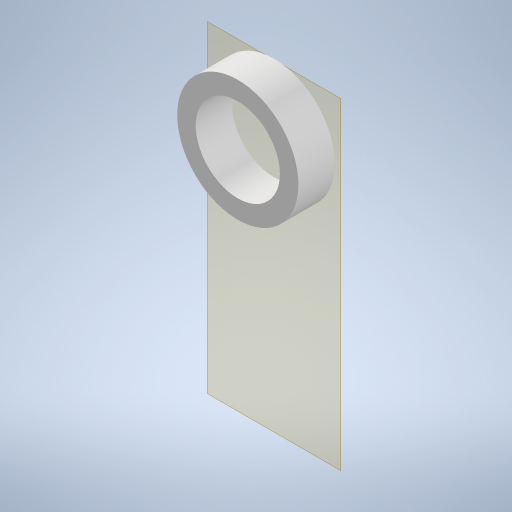
# Autodesk Inventor part: spacerA_V3
Saved by Autodesk Inventor 2023 (Build 270158000, 158)
## iProperties
Created: 2022-11-25
Part Number: spacerA_V3
Material: Generic
Document SubType Name: Modeling
Designer: shrey
Density: 1 g/cm^3
Appearance: Default
Author: shrey
Autodesk Inventor part; units mm, degrees
(part 1 of 2)
ref_plane "YZ Plane" through (0, 0, 0) normal (1, 0, 0) x (0, 1, 0)
ref_plane "XZ Plane" through (0, 0, 0) normal (0, 1, 0) x (-1, 0, 0)
ref_plane "XY Plane" through (0, 0, 0) normal (0, 0, 1) x (1, 0, 0)
ref_plane "Work Plane1" through (-7.7432, -45.9796, 22.0468) normal (0, 0, 1) x (1, 0, 0)
sketch "Sketch1" plane through (-7.7432, -45.9796, 22.0468) normal (0, 0, 1) x (1, 0, 0)
  spline S0 degree 3 poles (3.2142, 51.1538) (3.1859, 51.0451) (3.1294, 50.8276) (3.0543, 50.4989) (2.9867, 50.1686) (2.9278, 49.8367) (2.8779, 49.5033) (2.8377, 49.1686) (2.808, 48.8328) (2.7898, 48.4962) (2.7854, 48.2152) (2.7893, 47.9905) (2.7963, 47.8221) (2.8075, 47.6539) (2.8251, 47.4863) (2.8413, 47.3468) (2.8467, 47.2345) (2.846, 47.1502) (2.8418, 47.066) (2.8328, 46.9822) (2.8184, 46.8991) (2.7981, 46.8172) (2.7715, 46.7372) (2.7385, 46.6595) (2.6988, 46.5851) (2.6518, 46.5149) (2.5985, 46.4496) (2.5398, 46.389) (2.4742, 46.3358) (2.4039, 46.2892) (2.3294, 46.2495) (2.2239, 46.2102) (2.0895, 46.1697) (1.9569, 46.1234) (1.8485, 46.0931) (1.7649, 46.0814) (1.6806, 46.0777) (1.5963, 46.0822) (1.5132, 46.0968) (1.4316, 46.1182) (1.3524, 46.1473) (1.2765, 46.1842) (1.2041, 46.2275) (1.1356, 46.2767) (1.071, 46.3309) (1.0104, 46.3896) (0.9538, 46.4521) (0.901, 46.5178) (0.8509, 46.5856) (0.7892, 46.6795) (0.7202, 46.8019) (0.6359, 46.9478) (0.546, 47.0905) (0.4527, 47.2308) (0.3236, 47.4148) (0.1549, 47.6395) (-0.0578, 47.901) (-0.2793, 48.1552) (-0.5087, 48.4022) (-0.7451, 48.6425) (-0.988, 48.8763) (-1.2369, 49.1037) (-1.4909, 49.3254) (-1.6645, 49.468) (-1.7513, 49.5393) knots -1.078574 -1.078574 -1.078574 -1.078574 -1.044867 -1.011159 -0.977452 -0.943745 -0.910038 -0.876331 -0.842624 -0.808918 -0.775212 -0.758359 -0.741505 -0.724651 -0.707798 -0.690947 -0.68252 -0.674093 -0.665668 -0.657242 -0.648815 -0.640389 -0.631963 -0.623537 -0.61511 -0.606685 -0.598264 -0.589839 -0.581413 -0.57299 -0.564565 -0.556141 -0.539287 -0.522433 -0.514009 -0.505584 -0.49716 -0.488735 -0.48031 -0.471889 -0.463464 -0.455037 -0.446611 -0.438185 -0.429758 -0.421332 -0.412906 -0.40448 -0.396053 -0.387627 -0.370775 -0.353922 -0.337069 -0.320215 -0.303361 -0.269656 -0.235949 -0.202243 -0.168536 -0.134829 -0.101122 -0.067415 -0.033707 0 0 0 0 construction
  arc A0 (-1.7513, 49.5393) -> (-3.0984, 48.9393) centre (10.5928, 20.0161) ccw construction
  spline S1 degree 3 poles (-3.0984, 48.9393) (-3.1035, 48.827) (-3.1136, 48.6025) (-3.1187, 48.2654) (-3.1161, 47.9283) (-3.1047, 47.5914) (-3.0843, 47.2549) (-3.054, 46.9192) (-3.0132, 46.5845) (-2.961, 46.2515) (-2.9069, 45.9757) (-2.8564, 45.7568) (-2.8145, 45.5935) (-2.7686, 45.4313) (-2.7165, 45.271) (-2.6717, 45.1379) (-2.6431, 45.0292) (-2.6262, 44.9466) (-2.6128, 44.8634) (-2.6041, 44.7795) (-2.601, 44.6952) (-2.6039, 44.6109) (-2.6132, 44.5271) (-2.6293, 44.4443) (-2.6527, 44.3632) (-2.6841, 44.2849) (-2.7227, 44.2099) (-2.7674, 44.1383) (-2.8205, 44.0727) (-2.8796, 44.0125) (-2.9443, 43.9582) (-3.0393, 43.8979) (-3.1623, 43.8302) (-3.2824, 43.7574) (-3.3821, 43.7052) (-3.4615, 43.6764) (-3.5432, 43.6553) (-3.6266, 43.6421) (-3.7109, 43.6391) (-3.7951, 43.6431) (-3.8787, 43.6551) (-3.9606, 43.6753) (-4.0404, 43.7027) (-4.1177, 43.7366) (-4.1921, 43.7762) (-4.2635, 43.821) (-4.3319, 43.8704) (-4.3973, 43.9236) (-4.4604, 43.9795) (-4.5403, 44.0586) (-4.6332, 44.164) (-4.746, 44.2892) (-4.8635, 44.41) (-4.984, 44.5279) (-5.1485, 44.681) (-5.3603, 44.8656) (-5.6227, 45.0773) (-5.8922, 45.2798) (-6.1679, 45.4738) (-6.4491, 45.6597) (-6.7353, 45.8379) (-7.026, 46.0085) (-7.3205, 46.1726) (-7.5201, 46.276) (-7.6198, 46.3277) knots -1.078574 -1.078574 -1.078574 -1.078574 -1.044867 -1.011159 -0.977452 -0.943745 -0.910038 -0.876331 -0.842624 -0.808918 -0.775212 -0.758359 -0.741505 -0.724651 -0.707798 -0.690947 -0.68252 -0.674093 -0.665668 -0.657242 -0.648815 -0.640389 -0.631963 -0.623537 -0.61511 -0.606685 -0.598264 -0.589839 -0.581413 -0.57299 -0.564565 -0.556141 -0.539287 -0.522433 -0.514009 -0.505584 -0.49716 -0.488735 -0.48031 -0.471889 -0.463464 -0.455037 -0.446611 -0.438185 -0.429758 -0.421332 -0.412906 -0.40448 -0.396053 -0.387627 -0.370775 -0.353922 -0.337069 -0.320215 -0.303361 -0.269656 -0.235949 -0.202243 -0.168536 -0.134829 -0.101122 -0.067415 -0.033707 0 0 0 0 construction
  arc A1 (-7.6198, 46.3277) -> (-8.8127, 45.4607) centre (10.5928, 20.0161) ccw construction
  spline S2 degree 3 poles (-8.8127, 45.4607) (-8.7943, 45.3498) (-8.7575, 45.1281) (-8.6924, 44.7973) (-8.6198, 44.4682) (-8.5387, 44.141) (-8.4487, 43.8161) (-8.3492, 43.494) (-8.2398, 43.1751) (-8.1195, 42.8602) (-8.0092, 42.6017) (-7.9143, 42.398) (-7.8394, 42.247) (-7.7607, 42.0979) (-7.6765, 41.952) (-7.6049, 41.8311) (-7.5543, 41.7307) (-7.5207, 41.6534) (-7.4902, 41.5748) (-7.4644, 41.4946) (-7.4438, 41.4128) (-7.429, 41.3297) (-7.4207, 41.2458) (-7.4193, 41.1614) (-7.4253, 41.0773) (-7.4397, 40.9941) (-7.4619, 40.9128) (-7.4908, 40.8335) (-7.529, 40.7582) (-7.5743, 40.687) (-7.6263, 40.6205) (-7.7067, 40.5417) (-7.813, 40.45) (-7.9153, 40.3538) (-8.002, 40.282) (-8.0736, 40.2373) (-8.1491, 40.1997) (-8.228, 40.1694) (-8.3098, 40.149) (-8.3931, 40.1354) (-8.4773, 40.1297) (-8.5616, 40.1325) (-8.6453, 40.1427) (-8.728, 40.1597) (-8.809, 40.183) (-8.8882, 40.212) (-8.9653, 40.2461) (-9.0403, 40.2846) (-9.1137, 40.3261) (-9.2083, 40.3868) (-9.3211, 40.4706) (-9.4575, 40.5696) (-9.5975, 40.6634) (-9.7399, 40.7536) (-9.9326, 40.8692) (-10.1782, 41.0058) (-10.4788, 41.1583) (-10.7846, 41.3003) (-11.0946, 41.4327) (-11.4083, 41.5561) (-11.7253, 41.6709) (-12.0451, 41.7774) (-12.3673, 41.8766) (-12.584, 41.9363) (-12.6923, 41.9661) knots -1.078574 -1.078574 -1.078574 -1.078574 -1.044867 -1.011159 -0.977452 -0.943745 -0.910038 -0.876331 -0.842624 -0.808918 -0.775212 -0.758359 -0.741505 -0.724651 -0.707798 -0.690947 -0.68252 -0.674093 -0.665668 -0.657242 -0.648815 -0.640389 -0.631963 -0.623537 -0.61511 -0.606685 -0.598264 -0.589839 -0.581413 -0.57299 -0.564565 -0.556141 -0.539287 -0.522433 -0.514009 -0.505584 -0.49716 -0.488735 -0.48031 -0.471889 -0.463464 -0.455037 -0.446611 -0.438185 -0.429758 -0.421332 -0.412906 -0.40448 -0.396053 -0.387627 -0.370775 -0.353922 -0.337069 -0.320215 -0.303361 -0.269656 -0.235949 -0.202243 -0.168536 -0.134829 -0.101122 -0.067415 -0.033707 0 0 0 0 construction
  arc A2 (-12.6923, 41.9661) -> (-13.6789, 40.87) centre (10.5928, 20.0161) ccw construction
  spline S3 degree 3 poles (-13.6789, 40.87) (-13.6378, 40.7654) (-13.5558, 40.5562) (-13.4233, 40.2462) (-13.2838, 39.9393) (-13.1364, 39.6361) (-12.9808, 39.337) (-12.8166, 39.0426) (-12.6433, 38.7535) (-12.4601, 38.4705) (-12.2985, 38.2406) (-12.1634, 38.0611) (-12.0587, 37.929) (-11.9507, 37.7995) (-11.838, 37.6742) (-11.7428, 37.5709) (-11.6725, 37.4832) (-11.6235, 37.4146) (-11.5774, 37.344) (-11.5354, 37.2709) (-11.4983, 37.1952) (-11.4666, 37.117) (-11.441, 37.0366) (-11.4221, 36.9544) (-11.4104, 36.8709) (-11.4072, 36.7865) (-11.412, 36.7023) (-11.4238, 36.6188) (-11.4456, 36.5372) (-11.4751, 36.4582) (-11.512, 36.3822) (-11.5743, 36.2885) (-11.6592, 36.1766) (-11.7393, 36.0613) (-11.8092, 35.9731) (-11.87, 35.9144) (-11.936, 35.8619) (-12.0068, 35.816) (-12.0826, 35.7789) (-12.1612, 35.7483) (-12.2424, 35.7253) (-12.3255, 35.7105) (-12.4095, 35.7031) (-12.4939, 35.7025) (-12.578, 35.7085) (-12.6615, 35.7204) (-12.744, 35.7377) (-12.8254, 35.7597) (-12.9057, 35.7851) (-13.0109, 35.8248) (-13.1386, 35.8833) (-13.2926, 35.9518) (-13.4491, 36.0144) (-13.6071, 36.0731) (-13.8197, 36.1461) (-14.0883, 36.2286) (-14.4141, 36.3152) (-14.7427, 36.3906) (-15.0734, 36.4557) (-15.406, 36.5111) (-15.7399, 36.5575) (-16.0749, 36.5951) (-16.4106, 36.6252) (-16.635, 36.6385) (-16.7471, 36.6452) knots -1.078574 -1.078574 -1.078574 -1.078574 -1.044867 -1.011159 -0.977452 -0.943745 -0.910038 -0.876331 -0.842624 -0.808918 -0.775212 -0.758359 -0.741505 -0.724651 -0.707798 -0.690947 -0.68252 -0.674093 -0.665668 -0.657242 -0.648815 -0.640389 -0.631963 -0.623537 -0.61511 -0.606685 -0.598264 -0.589839 -0.581413 -0.57299 -0.564565 -0.556141 -0.539287 -0.522433 -0.514009 -0.505584 -0.49716 -0.488735 -0.48031 -0.471889 -0.463464 -0.455037 -0.446611 -0.438185 -0.429758 -0.421332 -0.412906 -0.40448 -0.396053 -0.387627 -0.370775 -0.353922 -0.337069 -0.320215 -0.303361 -0.269656 -0.235949 -0.202243 -0.168536 -0.134829 -0.101122 -0.067415 -0.033707 0 0 0 0 construction
  arc A3 (-16.7471, 36.6452) -> (-17.4843, 35.3679) centre (10.5928, 20.0161) ccw construction
  spline S4 degree 3 poles (-17.4843, 35.3679) (-17.4224, 35.2741) (-17.2986, 35.0866) (-17.1045, 34.8109) (-16.9043, 34.5397) (-16.6971, 34.2738) (-16.4828, 34.0136) (-16.2609, 33.7598) (-16.0312, 33.513) (-15.7932, 33.2742) (-15.5874, 33.083) (-15.4178, 32.9355) (-15.288, 32.828) (-15.1555, 32.7238) (-15.0191, 32.6247) (-14.9046, 32.5434) (-14.8176, 32.4722) (-14.7554, 32.4154) (-14.6956, 32.3559) (-14.6393, 32.2931) (-14.5872, 32.2268) (-14.54, 32.1569) (-14.4983, 32.0836) (-14.4627, 32.0071) (-14.4339, 31.9278) (-14.4132, 31.846) (-14.4004, 31.7626) (-14.3946, 31.6785) (-14.3989, 31.5941) (-14.4113, 31.5107) (-14.4317, 31.4287) (-14.4731, 31.3241) (-14.5329, 31.197) (-14.5873, 31.0675) (-14.6373, 30.9668) (-14.6845, 30.8967) (-14.7382, 30.8317) (-14.7979, 30.772) (-14.8644, 30.72) (-14.9349, 30.6737) (-15.0095, 30.6343) (-15.0877, 30.6026) (-15.1684, 30.5778) (-15.2507, 30.5597) (-15.3343, 30.5481) (-15.4184, 30.5423) (-15.5027, 30.5421) (-15.5869, 30.5467) (-15.6708, 30.5549) (-15.7819, 30.5719) (-15.919, 30.6025) (-16.0839, 30.6375) (-16.25, 30.6662) (-16.4167, 30.6907) (-16.6398, 30.718) (-16.9197, 30.7428) (-17.2564, 30.7598) (-17.5935, 30.7652) (-17.9306, 30.7601) (-18.2673, 30.7452) (-18.6036, 30.7211) (-18.9391, 30.6883) (-19.2738, 30.6479) (-19.496, 30.6143) (-19.6071, 30.5975) knots -1.078574 -1.078574 -1.078574 -1.078574 -1.044867 -1.011159 -0.977452 -0.943745 -0.910038 -0.876331 -0.842624 -0.808918 -0.775212 -0.758359 -0.741505 -0.724651 -0.707798 -0.690947 -0.68252 -0.674093 -0.665668 -0.657242 -0.648815 -0.640389 -0.631963 -0.623537 -0.61511 -0.606685 -0.598264 -0.589839 -0.581413 -0.57299 -0.564565 -0.556141 -0.539287 -0.522433 -0.514009 -0.505584 -0.49716 -0.488735 -0.48031 -0.471889 -0.463464 -0.455037 -0.446611 -0.438185 -0.429758 -0.421332 -0.412906 -0.40448 -0.396053 -0.387627 -0.370775 -0.353922 -0.337069 -0.320215 -0.303361 -0.269656 -0.235949 -0.202243 -0.168536 -0.134829 -0.101122 -0.067415 -0.033707 0 0 0 0 construction
  arc A4 (-19.6071, 30.5975) -> (-20.0625, 29.1949) centre (10.5928, 20.0161) ccw construction
  spline S5 degree 3 poles (-20.0625, 29.1949) (-19.9825, 29.116) (-19.8224, 28.9583) (-19.5753, 28.729) (-19.3231, 28.5053) (-19.0651, 28.2883) (-18.8013, 28.0784) (-18.5316, 27.8762) (-18.2556, 27.6826) (-17.9731, 27.4985) (-17.732, 27.3542) (-17.5355, 27.2452) (-17.3862, 27.1671) (-17.2349, 27.0927) (-17.0809, 27.0242) (-16.952, 26.9684) (-16.8521, 26.9169) (-16.7794, 26.8742) (-16.7086, 26.8285) (-16.6405, 26.7788) (-16.5757, 26.7247) (-16.515, 26.6662) (-16.4589, 26.6032) (-16.4082, 26.5358) (-16.3636, 26.4642) (-16.3264, 26.3884) (-16.2965, 26.3096) (-16.2733, 26.2284) (-16.26, 26.1451) (-16.2548, 26.0609) (-16.2577, 25.9765) (-16.2764, 25.8655) (-16.3085, 25.7288) (-16.3348, 25.5908) (-16.3627, 25.4818) (-16.3944, 25.4035) (-16.4333, 25.3287) (-16.4794, 25.2579) (-16.5335, 25.1932) (-16.5929, 25.1333) (-16.6577, 25.0793) (-16.7276, 25.0319) (-16.8013, 24.991) (-16.8781, 24.9562) (-16.9574, 24.9274) (-17.0385, 24.9043) (-17.121, 24.8865) (-17.2042, 24.8735) (-17.288, 24.8641) (-17.4002, 24.8576) (-17.5407, 24.8591) (-17.7092, 24.859) (-17.8777, 24.8525) (-18.0459, 24.8418) (-18.2698, 24.8221) (-18.5487, 24.7882) (-18.8816, 24.7349) (-19.2124, 24.6701) (-19.5411, 24.595) (-19.8674, 24.5104) (-20.1913, 24.4169) (-20.5126, 24.3151) (-20.8316, 24.206) (-21.042, 24.1269) (-21.1471, 24.0874) knots -1.078574 -1.078574 -1.078574 -1.078574 -1.044867 -1.011159 -0.977452 -0.943745 -0.910038 -0.876331 -0.842624 -0.808918 -0.775212 -0.758359 -0.741505 -0.724651 -0.707798 -0.690947 -0.68252 -0.674093 -0.665668 -0.657242 -0.648815 -0.640389 -0.631963 -0.623537 -0.61511 -0.606685 -0.598264 -0.589839 -0.581413 -0.57299 -0.564565 -0.556141 -0.539287 -0.522433 -0.514009 -0.505584 -0.49716 -0.488735 -0.48031 -0.471889 -0.463464 -0.455037 -0.446611 -0.438185 -0.429758 -0.421332 -0.412906 -0.40448 -0.396053 -0.387627 -0.370775 -0.353922 -0.337069 -0.320215 -0.303361 -0.269656 -0.235949 -0.202243 -0.168536 -0.134829 -0.101122 -0.067415 -0.033707 0 0 0 0 construction
  arc A5 (-21.1471, 24.0874) -> (-21.301, 22.6207) centre (10.5928, 20.0161) ccw construction
  spline S6 degree 3 poles (-21.301, 22.6207) (-21.2063, 22.5602) (-21.017, 22.4392) (-20.7276, 22.2663) (-20.4344, 22.1) (-20.1369, 21.9413) (-19.8352, 21.7908) (-19.5293, 21.6492) (-19.2191, 21.5171) (-18.9046, 21.3958) (-18.6388, 21.3048) (-18.4239, 21.239) (-18.2615, 21.1937) (-18.0981, 21.1524) (-17.9333, 21.1174) (-17.7955, 21.0896) (-17.6871, 21.06) (-17.6071, 21.0334) (-17.5283, 21.0034) (-17.4514, 20.9689) (-17.3768, 20.9295) (-17.3053, 20.8849) (-17.2373, 20.8349) (-17.1737, 20.7795) (-17.1152, 20.7187) (-17.063, 20.6524) (-17.0174, 20.5814) (-16.9778, 20.5069) (-16.9475, 20.4281) (-16.9249, 20.3469) (-16.9102, 20.2637) (-16.9054, 20.1513) (-16.9084, 20.0108) (-16.9054, 19.8704) (-16.9101, 19.758) (-16.9248, 19.6748) (-16.9473, 19.5936) (-16.9776, 19.5148) (-17.0172, 19.4402) (-17.0627, 19.3693) (-17.1149, 19.3029) (-17.1734, 19.2421) (-17.237, 19.1867) (-17.3049, 19.1367) (-17.3765, 19.092) (-17.451, 19.0526) (-17.528, 19.0181) (-17.6067, 18.9881) (-17.6867, 18.9614) (-17.7951, 18.9317) (-17.9328, 18.9039) (-18.0977, 18.8688) (-18.2611, 18.8275) (-18.4234, 18.7821) (-18.6383, 18.7162) (-18.9041, 18.6251) (-19.2186, 18.5037) (-19.5287, 18.3715) (-19.8346, 18.2297) (-20.1362, 18.0791) (-20.4336, 17.9204) (-20.7267, 17.7539) (-21.016, 17.5809) (-21.2054, 17.4598) (-21.3, 17.3993) knots -1.078574 -1.078574 -1.078574 -1.078574 -1.044867 -1.011159 -0.977452 -0.943745 -0.910038 -0.876331 -0.842624 -0.808918 -0.775212 -0.758359 -0.741505 -0.724651 -0.707798 -0.690947 -0.68252 -0.674093 -0.665668 -0.657242 -0.648815 -0.640389 -0.631963 -0.623537 -0.61511 -0.606685 -0.598264 -0.589839 -0.581413 -0.57299 -0.564565 -0.556141 -0.539287 -0.522433 -0.514009 -0.505584 -0.49716 -0.488735 -0.48031 -0.471889 -0.463464 -0.455037 -0.446611 -0.438185 -0.429758 -0.421332 -0.412906 -0.40448 -0.396053 -0.387627 -0.370775 -0.353922 -0.337069 -0.320215 -0.303361 -0.269656 -0.235949 -0.202243 -0.168536 -0.134829 -0.101122 -0.067415 -0.033707 0 0 0 0 construction
  arc A6 (-21.3, 17.3993) -> (-21.1456, 15.9327) centre (10.5928, 20.0161) ccw construction
  spline S7 degree 3 poles (-21.1456, 15.9327) (-21.0404, 15.8932) (-20.83, 15.8142) (-20.511, 15.7052) (-20.1896, 15.6035) (-19.8657, 15.5102) (-19.5393, 15.4257) (-19.2106, 15.3507) (-18.8798, 15.2861) (-18.5469, 15.2328) (-18.2679, 15.1991) (-18.0441, 15.1794) (-17.8758, 15.1688) (-17.7074, 15.1624) (-17.5389, 15.1624) (-17.3984, 15.1639) (-17.2861, 15.1575) (-17.2024, 15.148) (-17.1191, 15.1351) (-17.0367, 15.1174) (-16.9555, 15.0943) (-16.8763, 15.0655) (-16.7994, 15.0308) (-16.7256, 14.9898) (-16.6558, 14.9425) (-16.5909, 14.8885) (-16.5316, 14.8286) (-16.4773, 14.7639) (-16.4313, 14.6932) (-16.3923, 14.6184) (-16.3606, 14.5401) (-16.3326, 14.4311) (-16.3063, 14.2931) (-16.2742, 14.1564) (-16.2554, 14.0455) (-16.2525, 13.9611) (-16.2576, 13.8769) (-16.2709, 13.7935) (-16.2941, 13.7124) (-16.3239, 13.6335) (-16.3611, 13.5578) (-16.4057, 13.4861) (-16.4564, 13.4187) (-16.5125, 13.3556) (-16.5732, 13.2971) (-16.6379, 13.243) (-16.706, 13.1933) (-16.7768, 13.1475) (-16.8494, 13.1048) (-16.9493, 13.0532) (-17.0783, 12.9974) (-17.2322, 12.9288) (-17.3834, 12.8544) (-17.5328, 12.7762) (-17.7292, 12.6671) (-17.9703, 12.5228) (-18.2527, 12.3386) (-18.5286, 12.1449) (-18.7983, 11.9426) (-19.0619, 11.7325) (-19.3198, 11.5154) (-19.572, 11.2917) (-19.819, 11.0623) (-19.979, 10.9045) (-20.059, 10.8256) knots -1.078574 -1.078574 -1.078574 -1.078574 -1.044867 -1.011159 -0.977452 -0.943745 -0.910038 -0.876331 -0.842624 -0.808918 -0.775212 -0.758359 -0.741505 -0.724651 -0.707798 -0.690947 -0.68252 -0.674093 -0.665668 -0.657242 -0.648815 -0.640389 -0.631963 -0.623537 -0.61511 -0.606685 -0.598264 -0.589839 -0.581413 -0.57299 -0.564565 -0.556141 -0.539287 -0.522433 -0.514009 -0.505584 -0.49716 -0.488735 -0.48031 -0.471889 -0.463464 -0.455037 -0.446611 -0.438185 -0.429758 -0.421332 -0.412906 -0.40448 -0.396053 -0.387627 -0.370775 -0.353922 -0.337069 -0.320215 -0.303361 -0.269656 -0.235949 -0.202243 -0.168536 -0.134829 -0.101122 -0.067415 -0.033707 0 0 0 0 construction
  arc A7 (-20.059, 10.8256) -> (-19.603, 9.4231) centre (10.5928, 20.0161) ccw construction
  spline S8 degree 3 poles (-19.603, 9.4231) (-19.4919, 9.4064) (-19.2697, 9.3729) (-18.935, 9.3326) (-18.5995, 9.2999) (-18.2632, 9.276) (-17.9264, 9.2612) (-17.5894, 9.2562) (-17.2523, 9.2618) (-16.9156, 9.2789) (-16.6357, 9.3038) (-16.4127, 9.3312) (-16.2459, 9.3558) (-16.0798, 9.3845) (-15.915, 9.4196) (-15.7779, 9.4502) (-15.6668, 9.4673) (-15.5829, 9.4755) (-15.4987, 9.4801) (-15.4144, 9.4799) (-15.3302, 9.4742) (-15.2467, 9.4626) (-15.1643, 9.4445) (-15.0836, 9.4198) (-15.0055, 9.3881) (-14.9308, 9.3487) (-14.8603, 9.3025) (-14.7938, 9.2505) (-14.7341, 9.1909) (-14.6804, 9.1258) (-14.6331, 9.0558) (-14.5831, 8.955) (-14.5286, 8.8256) (-14.4688, 8.6985) (-14.4273, 8.5939) (-14.4069, 8.5119) (-14.3945, 8.4285) (-14.3901, 8.3442) (-14.3959, 8.26) (-14.4087, 8.1767) (-14.4294, 8.0948) (-14.4581, 8.0155) (-14.4936, 7.939) (-14.5354, 7.8657) (-14.5826, 7.7958) (-14.6346, 7.7294) (-14.6909, 7.6666) (-14.7506, 7.6072) (-14.8128, 7.5503) (-14.8998, 7.4791) (-15.0143, 7.3977) (-15.1506, 7.2986) (-15.2831, 7.1943) (-15.4129, 7.0868) (-15.5824, 6.9392) (-15.7882, 6.7479) (-16.0261, 6.5091) (-16.2557, 6.2622) (-16.4774, 6.0083) (-16.6917, 5.748) (-16.8988, 5.482) (-17.0989, 5.2107) (-17.2928, 4.935) (-17.4165, 4.7474) (-17.4784, 4.6536) knots -1.078574 -1.078574 -1.078574 -1.078574 -1.044867 -1.011159 -0.977452 -0.943745 -0.910038 -0.876331 -0.842624 -0.808918 -0.775212 -0.758359 -0.741505 -0.724651 -0.707798 -0.690947 -0.68252 -0.674093 -0.665668 -0.657242 -0.648815 -0.640389 -0.631963 -0.623537 -0.61511 -0.606685 -0.598264 -0.589839 -0.581413 -0.57299 -0.564565 -0.556141 -0.539287 -0.522433 -0.514009 -0.505584 -0.49716 -0.488735 -0.48031 -0.471889 -0.463464 -0.455037 -0.446611 -0.438185 -0.429758 -0.421332 -0.412906 -0.40448 -0.396053 -0.387627 -0.370775 -0.353922 -0.337069 -0.320215 -0.303361 -0.269656 -0.235949 -0.202243 -0.168536 -0.134829 -0.101122 -0.067415 -0.033707 0 0 0 0 construction
  arc A8 (-17.4784, 4.6536) -> (-16.7408, 3.3766) centre (10.5928, 20.0161) ccw construction
  spline S9 degree 3 poles (-16.7408, 3.3766) (-16.6286, 3.3833) (-16.4043, 3.3967) (-16.0685, 3.4269) (-15.7336, 3.4647) (-15.3997, 3.5112) (-15.0672, 3.5667) (-14.7364, 3.6319) (-14.4078, 3.7074) (-14.0821, 3.7942) (-13.8135, 3.8768) (-13.601, 3.9499) (-13.443, 4.0086) (-13.2865, 4.0713) (-13.1326, 4.1398) (-13.0048, 4.1984) (-12.8997, 4.2381) (-12.8193, 4.2636) (-12.738, 4.2856) (-12.6555, 4.303) (-12.572, 4.3149) (-12.4879, 4.3209) (-12.4035, 4.3204) (-12.3195, 4.313) (-12.2364, 4.2982) (-12.1552, 4.2752) (-12.0766, 4.2446) (-12.0008, 4.2076) (-11.9299, 4.1617) (-11.8639, 4.1092) (-11.8031, 4.0506) (-11.7332, 3.9624) (-11.653, 3.8471) (-11.5681, 3.7352) (-11.5058, 3.6415) (-11.4688, 3.5656) (-11.4392, 3.4866) (-11.4174, 3.405) (-11.4056, 3.3215) (-11.4008, 3.2373) (-11.404, 3.1529) (-11.4156, 3.0694) (-11.4345, 2.9871) (-11.46, 2.9068) (-11.4917, 2.8286) (-11.5288, 2.7528) (-11.5708, 2.6797) (-11.6168, 2.6091) (-11.6658, 2.5405) (-11.7361, 2.4528) (-11.8312, 2.3494) (-11.9439, 2.2241) (-12.0518, 2.0946) (-12.1565, 1.9624) (-12.2916, 1.7829) (-12.4531, 1.5529) (-12.6361, 1.2698) (-12.8094, 0.9806) (-12.9735, 0.6861) (-13.1289, 0.387) (-13.2762, 0.0838) (-13.4155, -0.2232) (-13.5479, -0.5332) (-13.6299, -0.7424) (-13.6709, -0.8471) knots -1.078574 -1.078574 -1.078574 -1.078574 -1.044867 -1.011159 -0.977452 -0.943745 -0.910038 -0.876331 -0.842624 -0.808918 -0.775212 -0.758359 -0.741505 -0.724651 -0.707798 -0.690947 -0.68252 -0.674093 -0.665668 -0.657242 -0.648815 -0.640389 -0.631963 -0.623537 -0.61511 -0.606685 -0.598264 -0.589839 -0.581413 -0.57299 -0.564565 -0.556141 -0.539287 -0.522433 -0.514009 -0.505584 -0.49716 -0.488735 -0.48031 -0.471889 -0.463464 -0.455037 -0.446611 -0.438185 -0.429758 -0.421332 -0.412906 -0.40448 -0.396053 -0.387627 -0.370775 -0.353922 -0.337069 -0.320215 -0.303361 -0.269656 -0.235949 -0.202243 -0.168536 -0.134829 -0.101122 -0.067415 -0.033707 0 0 0 0 construction
  arc A9 (-13.6709, -0.8471) -> (-12.6839, -1.9428) centre (10.5928, 20.0161) ccw construction
  spline S10 degree 3 poles (-12.6839, -1.9428) (-12.5756, -1.9129) (-12.359, -1.8532) (-12.0368, -1.7538) (-11.717, -1.6472) (-11.4001, -1.5323) (-11.0864, -1.4088) (-10.7764, -1.2763) (-10.4708, -1.1341) (-10.1701, -0.9815) (-9.9246, -0.8449) (-9.732, -0.7292) (-9.5896, -0.6389) (-9.4496, -0.5451) (-9.3132, -0.446) (-9.2005, -0.3622) (-9.1059, -0.3014) (-9.0326, -0.2599) (-8.9576, -0.2214) (-8.8805, -0.1872) (-8.8013, -0.1582) (-8.7203, -0.1349) (-8.6377, -0.1179) (-8.5539, -0.1076) (-8.4696, -0.1048) (-8.3854, -0.1104) (-8.3021, -0.124) (-8.2203, -0.1444) (-8.1414, -0.1746) (-8.0659, -0.2122) (-7.9943, -0.2569) (-7.9075, -0.3286) (-7.8052, -0.4248) (-7.6988, -0.5165) (-7.6184, -0.5952) (-7.5664, -0.6618) (-7.5211, -0.7329) (-7.4828, -0.8082) (-7.4539, -0.8874) (-7.4317, -0.9688) (-7.4173, -1.0519) (-7.4112, -1.1361) (-7.4126, -1.2205) (-7.4209, -1.3044) (-7.4356, -1.3875) (-7.4561, -1.4692) (-7.482, -1.5495) (-7.5124, -1.6281) (-7.546, -1.7054) (-7.5966, -1.8058) (-7.6681, -1.9268) (-7.7523, -2.0727) (-7.8309, -2.2219) (-7.9058, -2.3729) (-8.0006, -2.5766) (-8.1107, -2.8351) (-8.2309, -3.1501) (-8.3403, -3.469) (-8.4396, -3.7911) (-8.5294, -4.1161) (-8.6105, -4.4433) (-8.6829, -4.7725) (-8.7479, -5.1033) (-8.7846, -5.325) (-8.803, -5.4359) knots -1.078574 -1.078574 -1.078574 -1.078574 -1.044867 -1.011159 -0.977452 -0.943745 -0.910038 -0.876331 -0.842624 -0.808918 -0.775212 -0.758359 -0.741505 -0.724651 -0.707798 -0.690947 -0.68252 -0.674093 -0.665668 -0.657242 -0.648815 -0.640389 -0.631963 -0.623537 -0.61511 -0.606685 -0.598264 -0.589839 -0.581413 -0.57299 -0.564565 -0.556141 -0.539287 -0.522433 -0.514009 -0.505584 -0.49716 -0.488735 -0.48031 -0.471889 -0.463464 -0.455037 -0.446611 -0.438185 -0.429758 -0.421332 -0.412906 -0.40448 -0.396053 -0.387627 -0.370775 -0.353922 -0.337069 -0.320215 -0.303361 -0.269656 -0.235949 -0.202243 -0.168536 -0.134829 -0.101122 -0.067415 -0.033707 0 0 0 0 construction
  arc A10 (-8.803, -5.4359) -> (-7.6098, -6.3025) centre (10.5928, 20.0161) ccw construction
  spline S11 degree 3 poles (-7.6098, -6.3025) (-7.51, -6.2507) (-7.3105, -6.1472) (-7.0161, -5.983) (-6.7254, -5.8123) (-6.4393, -5.634) (-6.1582, -5.448) (-5.8825, -5.2539) (-5.6131, -5.0513) (-5.3508, -4.8395) (-5.139, -4.6548) (-4.9746, -4.5016) (-4.8542, -4.3837) (-4.7367, -4.2628) (-4.6239, -4.1376) (-4.5311, -4.0322) (-4.4512, -3.953) (-4.3881, -3.8971) (-4.3228, -3.8439) (-4.2544, -3.7945) (-4.183, -3.7496) (-4.1086, -3.71) (-4.0313, -3.6761) (-3.9516, -3.6487) (-3.8696, -3.6284) (-3.7861, -3.6164) (-3.7019, -3.6123) (-3.6175, -3.6153) (-3.5341, -3.6285) (-3.4525, -3.6495) (-3.3731, -3.6784) (-3.2734, -3.7305) (-3.1532, -3.8033) (-3.0301, -3.8709) (-2.9351, -3.9311) (-2.8704, -3.9854) (-2.8113, -4.0456) (-2.7582, -4.1112) (-2.7134, -4.1828) (-2.6748, -4.2577) (-2.6434, -4.3361) (-2.62, -4.4171) (-2.6038, -4.4999) (-2.5945, -4.5838) (-2.5916, -4.6681) (-2.5947, -4.7523) (-2.6033, -4.8362) (-2.6167, -4.9194) (-2.6335, -5.002) (-2.662, -5.1108) (-2.7069, -5.2439) (-2.7589, -5.4042) (-2.8048, -5.5664) (-2.8466, -5.7297) (-2.897, -5.9487) (-2.951, -6.2244) (-3.0031, -6.5575) (-3.0437, -6.8922) (-3.0738, -7.228) (-3.0942, -7.5645) (-3.1054, -7.9014) (-3.1079, -8.2385) (-3.1027, -8.5756) (-3.0925, -8.8) (-3.0874, -8.9123) knots -1.078574 -1.078574 -1.078574 -1.078574 -1.044867 -1.011159 -0.977452 -0.943745 -0.910038 -0.876331 -0.842624 -0.808918 -0.775212 -0.758359 -0.741505 -0.724651 -0.707798 -0.690947 -0.68252 -0.674093 -0.665668 -0.657242 -0.648815 -0.640389 -0.631963 -0.623537 -0.61511 -0.606685 -0.598264 -0.589839 -0.581413 -0.57299 -0.564565 -0.556141 -0.539287 -0.522433 -0.514009 -0.505584 -0.49716 -0.488735 -0.48031 -0.471889 -0.463464 -0.455037 -0.446611 -0.438185 -0.429758 -0.421332 -0.412906 -0.40448 -0.396053 -0.387627 -0.370775 -0.353922 -0.337069 -0.320215 -0.303361 -0.269656 -0.235949 -0.202243 -0.168536 -0.134829 -0.101122 -0.067415 -0.033707 0 0 0 0 construction
  arc A11 (-3.0874, -8.9123) -> (-1.7401, -9.5119) centre (10.5928, 20.0161) ccw construction
  spline S12 degree 3 poles (-1.7401, -9.5119) (-1.6533, -9.4405) (-1.4797, -9.2978) (-1.2258, -9.076) (-0.977, -8.8485) (-0.7342, -8.6147) (-0.4978, -8.3743) (-0.2686, -8.1271) (-0.0472, -7.8729) (0.1654, -7.6112) (0.3341, -7.3865) (0.4631, -7.2025) (0.5564, -7.0621) (0.6461, -6.9194) (0.7304, -6.7735) (0.7993, -6.6511) (0.861, -6.5571) (0.9111, -6.4893) (0.9639, -6.4236) (1.0205, -6.3611) (1.081, -6.3024) (1.1456, -6.2481) (1.2141, -6.1989) (1.2865, -6.1555) (1.3624, -6.1186) (1.4416, -6.0895) (1.5231, -6.068) (1.6062, -6.0534) (1.6906, -6.0489) (1.7748, -6.0526) (1.8585, -6.0643) (1.9668, -6.0945) (2.0995, -6.1407) (2.2339, -6.1812) (2.3394, -6.2204) (2.414, -6.2601) (2.4843, -6.3067) (2.5499, -6.3598) (2.6086, -6.4205) (2.662, -6.4858) (2.7089, -6.5559) (2.7487, -6.6303) (2.7817, -6.7079) (2.8083, -6.788) (2.8287, -6.8698) (2.8432, -6.9529) (2.8522, -7.0367) (2.8564, -7.1209) (2.8571, -7.2052) (2.8518, -7.3175) (2.8356, -7.4571) (2.8181, -7.6247) (2.8069, -7.7929) (2.7999, -7.9613) (2.7962, -8.186) (2.8007, -8.4669) (2.819, -8.8036) (2.8488, -9.1394) (2.8892, -9.4741) (2.9392, -9.8074) (2.9983, -10.1393) (3.066, -10.4696) (3.1411, -10.7982) (3.1978, -11.0157) (3.2261, -11.1244) knots -1.078574 -1.078574 -1.078574 -1.078574 -1.044867 -1.011159 -0.977452 -0.943745 -0.910038 -0.876331 -0.842624 -0.808918 -0.775212 -0.758359 -0.741505 -0.724651 -0.707798 -0.690947 -0.68252 -0.674093 -0.665668 -0.657242 -0.648815 -0.640389 -0.631963 -0.623537 -0.61511 -0.606685 -0.598264 -0.589839 -0.581413 -0.57299 -0.564565 -0.556141 -0.539287 -0.522433 -0.514009 -0.505584 -0.49716 -0.488735 -0.48031 -0.471889 -0.463464 -0.455037 -0.446611 -0.438185 -0.429758 -0.421332 -0.412906 -0.40448 -0.396053 -0.387627 -0.370775 -0.353922 -0.337069 -0.320215 -0.303361 -0.269656 -0.235949 -0.202243 -0.168536 -0.134829 -0.101122 -0.067415 -0.033707 0 0 0 0 construction
  arc A12 (3.2261, -11.1244) -> (4.6687, -11.4307) centre (10.5928, 20.0161) ccw construction
  spline S13 degree 3 poles (4.6687, -11.4307) (4.7387, -11.3429) (4.8789, -11.1672) (5.0811, -10.8975) (5.2772, -10.6233) (5.466, -10.344) (5.6472, -10.0598) (5.8201, -9.7703) (5.9838, -9.4756) (6.1373, -9.1755) (6.2556, -8.9206) (6.3435, -8.7138) (6.4056, -8.5571) (6.4637, -8.3989) (6.5158, -8.2386) (6.5578, -8.1045) (6.5986, -7.9998) (6.6334, -7.923) (6.6715, -7.8478) (6.7138, -7.7749) (6.7608, -7.7049) (6.8127, -7.6383) (6.8695, -7.576) (6.9312, -7.5185) (6.9978, -7.4667) (7.0692, -7.4217) (7.1445, -7.3837) (7.2228, -7.3522) (7.3043, -7.3302) (7.3875, -7.3163) (7.4717, -7.3103) (7.584, -7.3174) (7.7234, -7.335) (7.8633, -7.3467) (7.9747, -7.3631) (8.0558, -7.3864) (8.1343, -7.4173) (8.2095, -7.4557) (8.2795, -7.5028) (8.3453, -7.5556) (8.4058, -7.6144) (8.4602, -7.6789) (8.5087, -7.748) (8.5513, -7.8207) (8.5882, -7.8966) (8.6197, -7.9748) (8.6459, -8.0549) (8.6676, -8.1364) (8.6857, -8.2187) (8.7039, -8.3297) (8.7171, -8.4695) (8.7348, -8.6371) (8.7589, -8.804) (8.7871, -8.9701) (8.8301, -9.1907) (8.8929, -9.4646) (8.9808, -9.7901) (9.0798, -10.1123) (9.1889, -10.4313) (9.3071, -10.747) (9.4339, -11.0594) (9.5688, -11.3683) (9.7106, -11.6741) (9.8113, -11.8751) (9.8616, -11.9755) knots -1.078574 -1.078574 -1.078574 -1.078574 -1.044867 -1.011159 -0.977452 -0.943745 -0.910038 -0.876331 -0.842624 -0.808918 -0.775212 -0.758359 -0.741505 -0.724651 -0.707798 -0.690947 -0.68252 -0.674093 -0.665668 -0.657242 -0.648815 -0.640389 -0.631963 -0.623537 -0.61511 -0.606685 -0.598264 -0.589839 -0.581413 -0.57299 -0.564565 -0.556141 -0.539287 -0.522433 -0.514009 -0.505584 -0.49716 -0.488735 -0.48031 -0.471889 -0.463464 -0.455037 -0.446611 -0.438185 -0.429758 -0.421332 -0.412906 -0.40448 -0.396053 -0.387627 -0.370775 -0.353922 -0.337069 -0.320215 -0.303361 -0.269656 -0.235949 -0.202243 -0.168536 -0.134829 -0.101122 -0.067415 -0.033707 0 0 0 0 construction
  arc A13 (9.8616, -11.9755) -> (11.3363, -11.9753) centre (10.5928, 20.0161) ccw construction
  spline S14 degree 3 poles (11.3363, -11.9753) (11.3866, -11.8748) (11.4871, -11.6738) (11.6288, -11.3679) (11.7636, -11.0589) (11.8903, -10.7465) (12.0084, -10.4308) (12.1173, -10.1117) (12.2162, -9.7894) (12.304, -9.4639) (12.3667, -9.19) (12.4096, -8.9695) (12.4378, -8.8033) (12.4618, -8.6364) (12.4794, -8.4688) (12.4925, -8.3289) (12.5107, -8.218) (12.5288, -8.1357) (12.5504, -8.0542) (12.5766, -7.9741) (12.6081, -7.8958) (12.645, -7.82) (12.6876, -7.7472) (12.736, -7.6781) (12.7903, -7.6135) (12.8508, -7.5547) (12.9166, -7.5019) (12.9866, -7.4548) (13.0618, -7.4164) (13.1403, -7.3854) (13.2214, -7.3621) (13.3327, -7.3456) (13.4727, -7.3339) (13.612, -7.3162) (13.7243, -7.3091) (13.8086, -7.315) (13.8918, -7.329) (13.9733, -7.3509) (14.0516, -7.3824) (14.1269, -7.4203) (14.1983, -7.4653) (14.2649, -7.5171) (14.3267, -7.5746) (14.3835, -7.6369) (14.4354, -7.7034) (14.4824, -7.7734) (14.5248, -7.8463) (14.5629, -7.9215) (14.5978, -7.9982) (14.6386, -8.103) (14.6806, -8.237) (14.7328, -8.3973) (14.791, -8.5555) (14.8531, -8.7122) (14.9411, -8.919) (15.0594, -9.1738) (15.2131, -9.4739) (15.3769, -9.7685) (15.5499, -10.0579) (15.7312, -10.3421) (15.9202, -10.6212) (16.1164, -10.8954) (16.3187, -11.165) (16.4589, -11.3407) (16.529, -11.4285) knots -1.078574 -1.078574 -1.078574 -1.078574 -1.044867 -1.011159 -0.977452 -0.943745 -0.910038 -0.876331 -0.842624 -0.808918 -0.775212 -0.758359 -0.741505 -0.724651 -0.707798 -0.690947 -0.68252 -0.674093 -0.665668 -0.657242 -0.648815 -0.640389 -0.631963 -0.623537 -0.61511 -0.606685 -0.598264 -0.589839 -0.581413 -0.57299 -0.564565 -0.556141 -0.539287 -0.522433 -0.514009 -0.505584 -0.49716 -0.488735 -0.48031 -0.471889 -0.463464 -0.455037 -0.446611 -0.438185 -0.429758 -0.421332 -0.412906 -0.40448 -0.396053 -0.387627 -0.370775 -0.353922 -0.337069 -0.320215 -0.303361 -0.269656 -0.235949 -0.202243 -0.168536 -0.134829 -0.101122 -0.067415 -0.033707 0 0 0 0 construction
  arc A14 (16.529, -11.4285) -> (17.9714, -11.1216) centre (10.5928, 20.0161) ccw construction
  spline S15 degree 3 poles (17.9714, -11.1216) (17.9997, -11.0128) (18.0563, -10.7954) (18.1313, -10.4667) (18.1989, -10.1364) (18.2578, -9.8045) (18.3077, -9.4711) (18.3479, -9.1364) (18.3776, -8.8006) (18.3958, -8.4639) (18.4002, -8.183) (18.3964, -7.9583) (18.3893, -7.7899) (18.3781, -7.6217) (18.3605, -7.4541) (18.3443, -7.3145) (18.339, -7.2023) (18.3396, -7.118) (18.3438, -7.0338) (18.3528, -6.9499) (18.3672, -6.8669) (18.3876, -6.785) (18.4141, -6.7049) (18.4471, -6.6273) (18.4868, -6.5529) (18.5338, -6.4827) (18.5872, -6.4174) (18.6458, -6.3568) (18.7114, -6.3036) (18.7817, -6.257) (18.8562, -6.2173) (18.9617, -6.178) (19.0961, -6.1375) (19.2288, -6.0912) (19.3371, -6.0609) (19.4208, -6.0492) (19.505, -6.0455) (19.5893, -6.05) (19.6725, -6.0646) (19.754, -6.086) (19.8332, -6.1151) (19.9092, -6.1519) (19.9815, -6.1953) (20.0501, -6.2445) (20.1146, -6.2987) (20.1752, -6.3574) (20.2318, -6.4199) (20.2847, -6.4856) (20.3348, -6.5534) (20.3965, -6.6473) (20.4654, -6.7697) (20.5498, -6.9156) (20.6396, -7.0583) (20.733, -7.1986) (20.862, -7.3826) (21.0308, -7.6072) (21.2434, -7.8688) (21.4649, -8.123) (21.6943, -8.37) (21.9308, -8.6103) (22.1736, -8.8441) (22.4225, -9.0715) (22.6765, -9.2932) (22.8501, -9.4358) (22.937, -9.5071) knots -1.078574 -1.078574 -1.078574 -1.078574 -1.044867 -1.011159 -0.977452 -0.943745 -0.910038 -0.876331 -0.842624 -0.808918 -0.775212 -0.758359 -0.741505 -0.724651 -0.707798 -0.690947 -0.68252 -0.674093 -0.665668 -0.657242 -0.648815 -0.640389 -0.631963 -0.623537 -0.61511 -0.606685 -0.598264 -0.589839 -0.581413 -0.57299 -0.564565 -0.556141 -0.539287 -0.522433 -0.514009 -0.505584 -0.49716 -0.488735 -0.48031 -0.471889 -0.463464 -0.455037 -0.446611 -0.438185 -0.429758 -0.421332 -0.412906 -0.40448 -0.396053 -0.387627 -0.370775 -0.353922 -0.337069 -0.320215 -0.303361 -0.269656 -0.235949 -0.202243 -0.168536 -0.134829 -0.101122 -0.067415 -0.033707 0 0 0 0 construction
  arc A15 (22.937, -9.5071) -> (24.2841, -8.9071) centre (10.5928, 20.0161) ccw construction
  spline S16 degree 3 poles (24.2841, -8.9071) (24.2891, -8.7948) (24.2992, -8.5703) (24.3043, -8.2332) (24.3017, -7.8961) (24.2904, -7.5592) (24.2699, -7.2227) (24.2396, -6.887) (24.1989, -6.5523) (24.1466, -6.2193) (24.0925, -5.9435) (24.0421, -5.7246) (24.0002, -5.5613) (23.9542, -5.3991) (23.9021, -5.2388) (23.8573, -5.1057) (23.8287, -4.997) (23.8118, -4.9144) (23.7984, -4.8312) (23.7898, -4.7473) (23.7866, -4.663) (23.7895, -4.5787) (23.7988, -4.4949) (23.8149, -4.4121) (23.8383, -4.331) (23.8697, -4.2527) (23.9083, -4.1777) (23.9531, -4.1061) (24.0061, -4.0405) (24.0652, -3.9803) (24.1299, -3.926) (24.2249, -3.8656) (24.348, -3.798) (24.4681, -3.7252) (24.5678, -3.673) (24.6471, -3.6442) (24.7288, -3.6231) (24.8122, -3.6099) (24.8965, -3.6069) (24.9808, -3.6109) (25.0643, -3.6229) (25.1462, -3.6431) (25.226, -3.6705) (25.3033, -3.7043) (25.3777, -3.744) (25.4492, -3.7888) (25.5175, -3.8382) (25.5829, -3.8914) (25.646, -3.9473) (25.7259, -4.0264) (25.8188, -4.1318) (25.9316, -4.2569) (26.0491, -4.3778) (26.1696, -4.4957) (26.3341, -4.6488) (26.5459, -4.8334) (26.8083, -5.0451) (27.0778, -5.2476) (27.3535, -5.4416) (27.6348, -5.6275) (27.9209, -5.8057) (28.2117, -5.9763) (28.5062, -6.1404) (28.7057, -6.2438) (28.8054, -6.2955) knots -1.078574 -1.078574 -1.078574 -1.078574 -1.044867 -1.011159 -0.977452 -0.943745 -0.910038 -0.876331 -0.842624 -0.808918 -0.775212 -0.758359 -0.741505 -0.724651 -0.707798 -0.690947 -0.68252 -0.674093 -0.665668 -0.657242 -0.648815 -0.640389 -0.631963 -0.623537 -0.61511 -0.606685 -0.598264 -0.589839 -0.581413 -0.57299 -0.564565 -0.556141 -0.539287 -0.522433 -0.514009 -0.505584 -0.49716 -0.488735 -0.48031 -0.471889 -0.463464 -0.455037 -0.446611 -0.438185 -0.429758 -0.421332 -0.412906 -0.40448 -0.396053 -0.387627 -0.370775 -0.353922 -0.337069 -0.320215 -0.303361 -0.269656 -0.235949 -0.202243 -0.168536 -0.134829 -0.101122 -0.067415 -0.033707 0 0 0 0 construction
  arc A16 (28.8054, -6.2955) -> (29.9983, -5.4284) centre (10.5928, 20.0161) ccw construction
  spline S17 degree 3 poles (29.9983, -5.4284) (29.98, -5.3176) (29.9432, -5.0959) (29.878, -4.7651) (29.8054, -4.4359) (29.7243, -4.1088) (29.6343, -3.7839) (29.5349, -3.4617) (29.4254, -3.1429) (29.3051, -2.8279) (29.1949, -2.5695) (29.0999, -2.3658) (29.025, -2.2148) (28.9463, -2.0657) (28.8621, -1.9198) (28.7905, -1.7989) (28.74, -1.6985) (28.7063, -1.6212) (28.6758, -1.5426) (28.65, -1.4623) (28.6294, -1.3806) (28.6147, -1.2975) (28.6063, -1.2136) (28.6049, -1.1292) (28.6109, -1.0451) (28.6253, -0.9619) (28.6475, -0.8805) (28.6764, -0.8013) (28.7147, -0.726) (28.7599, -0.6548) (28.8119, -0.5882) (28.8923, -0.5095) (28.9986, -0.4177) (29.1009, -0.3216) (29.1876, -0.2498) (29.2593, -0.2051) (29.3347, -0.1675) (29.4136, -0.1372) (29.4955, -0.1167) (29.5787, -0.1032) (29.6629, -0.0975) (29.7472, -0.1003) (29.831, -0.1105) (29.9136, -0.1275) (29.9946, -0.1508) (30.0738, -0.1798) (30.151, -0.2139) (30.226, -0.2523) (30.2993, -0.2939) (30.3939, -0.3546) (30.5067, -0.4384) (30.6431, -0.5374) (30.7832, -0.6312) (30.9255, -0.7214) (31.1182, -0.837) (31.3638, -0.9736) (31.6645, -1.1261) (31.9702, -1.2681) (32.2802, -1.4005) (32.594, -1.5239) (32.9109, -1.6387) (33.2308, -1.7452) (33.553, -1.8444) (33.7696, -1.9041) (33.8779, -1.9339) knots -1.078574 -1.078574 -1.078574 -1.078574 -1.044867 -1.011159 -0.977452 -0.943745 -0.910038 -0.876331 -0.842624 -0.808918 -0.775212 -0.758359 -0.741505 -0.724651 -0.707798 -0.690947 -0.68252 -0.674093 -0.665668 -0.657242 -0.648815 -0.640389 -0.631963 -0.623537 -0.61511 -0.606685 -0.598264 -0.589839 -0.581413 -0.57299 -0.564565 -0.556141 -0.539287 -0.522433 -0.514009 -0.505584 -0.49716 -0.488735 -0.48031 -0.471889 -0.463464 -0.455037 -0.446611 -0.438185 -0.429758 -0.421332 -0.412906 -0.40448 -0.396053 -0.387627 -0.370775 -0.353922 -0.337069 -0.320215 -0.303361 -0.269656 -0.235949 -0.202243 -0.168536 -0.134829 -0.101122 -0.067415 -0.033707 0 0 0 0 construction
  arc A17 (33.8779, -1.9339) -> (34.8645, -0.8378) centre (10.5928, 20.0161) ccw construction
  spline S18 degree 3 poles (34.8645, -0.8378) (34.8235, -0.7332) (34.7414, -0.524) (34.6089, -0.214) (34.4695, 0.0929) (34.322, 0.3961) (34.1665, 0.6952) (34.0023, 0.9896) (33.8289, 1.2787) (33.6457, 1.5617) (33.4842, 1.7916) (33.349, 1.9711) (33.2443, 2.1032) (33.1363, 2.2327) (33.0236, 2.358) (32.9285, 2.4614) (32.8581, 2.5491) (32.8091, 2.6176) (32.763, 2.6882) (32.721, 2.7613) (32.6839, 2.837) (32.6522, 2.9152) (32.6266, 2.9956) (32.6077, 3.0778) (32.5961, 3.1614) (32.5928, 3.2457) (32.5976, 3.3299) (32.6094, 3.4134) (32.6312, 3.495) (32.6607, 3.574) (32.6977, 3.65) (32.7599, 3.7437) (32.8448, 3.8556) (32.9249, 3.9709) (32.9948, 4.0591) (33.0556, 4.1178) (33.1216, 4.1703) (33.1924, 4.2162) (33.2682, 4.2533) (33.3468, 4.2839) (33.428, 4.3069) (33.5111, 4.3217) (33.5951, 4.3291) (33.6795, 4.3297) (33.7636, 4.3237) (33.8471, 4.3119) (33.9296, 4.2945) (34.011, 4.2725) (34.0914, 4.2471) (34.1965, 4.2074) (34.3243, 4.1489) (34.4782, 4.0804) (34.6348, 4.0178) (34.7928, 3.9592) (35.0053, 3.8861) (35.2739, 3.8036) (35.5997, 3.717) (35.9283, 3.6416) (36.2591, 3.5765) (36.5916, 3.5211) (36.9255, 3.4747) (37.2605, 3.4371) (37.5963, 3.407) (37.8206, 3.3937) (37.9328, 3.387) knots -1.078574 -1.078574 -1.078574 -1.078574 -1.044867 -1.011159 -0.977452 -0.943745 -0.910038 -0.876331 -0.842624 -0.808918 -0.775212 -0.758359 -0.741505 -0.724651 -0.707798 -0.690947 -0.68252 -0.674093 -0.665668 -0.657242 -0.648815 -0.640389 -0.631963 -0.623537 -0.61511 -0.606685 -0.598264 -0.589839 -0.581413 -0.57299 -0.564565 -0.556141 -0.539287 -0.522433 -0.514009 -0.505584 -0.49716 -0.488735 -0.48031 -0.471889 -0.463464 -0.455037 -0.446611 -0.438185 -0.429758 -0.421332 -0.412906 -0.40448 -0.396053 -0.387627 -0.370775 -0.353922 -0.337069 -0.320215 -0.303361 -0.269656 -0.235949 -0.202243 -0.168536 -0.134829 -0.101122 -0.067415 -0.033707 0 0 0 0 construction
  arc A18 (37.9328, 3.387) -> (38.6699, 4.6643) centre (10.5928, 20.0161) ccw construction
  spline S19 degree 3 poles (38.6699, 4.6643) (38.608, 4.7581) (38.4842, 4.9456) (38.2902, 5.2213) (38.09, 5.4925) (37.8827, 5.7584) (37.6684, 6.0186) (37.4465, 6.2725) (37.2169, 6.5192) (36.9788, 6.758) (36.773, 6.9493) (36.6035, 7.0967) (36.4736, 7.2042) (36.3411, 7.3084) (36.2048, 7.4075) (36.0902, 7.4888) (36.0032, 7.56) (35.941, 7.6168) (35.8812, 7.6763) (35.8249, 7.7391) (35.7729, 7.8054) (35.7256, 7.8753) (35.6839, 7.9486) (35.6483, 8.0251) (35.6195, 8.1044) (35.5988, 8.1862) (35.586, 8.2696) (35.5802, 8.3538) (35.5845, 8.4381) (35.5969, 8.5215) (35.6173, 8.6035) (35.6587, 8.7081) (35.7185, 8.8352) (35.7729, 8.9647) (35.8229, 9.0655) (35.8702, 9.1355) (35.9238, 9.2005) (35.9835, 9.2602) (36.05, 9.3122) (36.1205, 9.3585) (36.1951, 9.3979) (36.2733, 9.4297) (36.354, 9.4544) (36.4364, 9.4725) (36.5199, 9.4841) (36.604, 9.4899) (36.6883, 9.4901) (36.7725, 9.4855) (36.8564, 9.4773) (36.9675, 9.4603) (37.1046, 9.4297) (37.2695, 9.3947) (37.4356, 9.366) (37.6024, 9.3415) (37.8254, 9.3143) (38.1053, 9.2894) (38.442, 9.2724) (38.7791, 9.267) (39.1162, 9.2721) (39.453, 9.287) (39.7892, 9.3111) (40.1247, 9.3439) (40.4594, 9.3843) (40.6816, 9.4179) (40.7927, 9.4347) knots -1.078574 -1.078574 -1.078574 -1.078574 -1.044867 -1.011159 -0.977452 -0.943745 -0.910038 -0.876331 -0.842624 -0.808918 -0.775212 -0.758359 -0.741505 -0.724651 -0.707798 -0.690947 -0.68252 -0.674093 -0.665668 -0.657242 -0.648815 -0.640389 -0.631963 -0.623537 -0.61511 -0.606685 -0.598264 -0.589839 -0.581413 -0.57299 -0.564565 -0.556141 -0.539287 -0.522433 -0.514009 -0.505584 -0.49716 -0.488735 -0.48031 -0.471889 -0.463464 -0.455037 -0.446611 -0.438185 -0.429758 -0.421332 -0.412906 -0.40448 -0.396053 -0.387627 -0.370775 -0.353922 -0.337069 -0.320215 -0.303361 -0.269656 -0.235949 -0.202243 -0.168536 -0.134829 -0.101122 -0.067415 -0.033707 0 0 0 0 construction
  arc A19 (40.7927, 9.4347) -> (41.2482, 10.8373) centre (10.5928, 20.0161) ccw construction
  spline S20 degree 3 poles (41.2482, 10.8373) (41.1681, 10.9162) (41.008, 11.0739) (40.7609, 11.3032) (40.5087, 11.5269) (40.2507, 11.7439) (39.987, 11.9538) (39.7172, 12.156) (39.4412, 12.3496) (39.1588, 12.5337) (38.9177, 12.678) (38.7211, 12.787) (38.5718, 12.8651) (38.4205, 12.9395) (38.2666, 13.008) (38.1376, 13.0638) (38.0377, 13.1153) (37.965, 13.158) (37.8942, 13.2037) (37.8261, 13.2534) (37.7614, 13.3075) (37.7006, 13.366) (37.6446, 13.429) (37.5938, 13.4964) (37.5492, 13.5681) (37.512, 13.6438) (37.4821, 13.7226) (37.4589, 13.8038) (37.4456, 13.8872) (37.4404, 13.9713) (37.4433, 14.0557) (37.462, 14.1667) (37.4941, 14.3034) (37.5204, 14.4414) (37.5483, 14.5504) (37.58, 14.6287) (37.619, 14.7035) (37.665, 14.7743) (37.7192, 14.839) (37.7785, 14.8989) (37.8433, 14.9529) (37.9132, 15.0003) (37.9869, 15.0412) (38.0638, 15.076) (38.143, 15.1048) (38.2241, 15.1279) (38.3066, 15.1457) (38.3899, 15.1587) (38.4736, 15.1681) (38.5858, 15.1746) (38.7263, 15.1731) (38.8949, 15.1732) (39.0633, 15.1797) (39.2315, 15.1904) (39.4554, 15.2101) (39.7343, 15.244) (40.0672, 15.2973) (40.398, 15.3621) (40.7267, 15.4372) (41.053, 15.5218) (41.3769, 15.6153) (41.6982, 15.7171) (42.0172, 15.8262) (42.2276, 15.9053) (42.3328, 15.9448) knots -1.078574 -1.078574 -1.078574 -1.078574 -1.044867 -1.011159 -0.977452 -0.943745 -0.910038 -0.876331 -0.842624 -0.808918 -0.775212 -0.758359 -0.741505 -0.724651 -0.707798 -0.690947 -0.68252 -0.674093 -0.665668 -0.657242 -0.648815 -0.640389 -0.631963 -0.623537 -0.61511 -0.606685 -0.598264 -0.589839 -0.581413 -0.57299 -0.564565 -0.556141 -0.539287 -0.522433 -0.514009 -0.505584 -0.49716 -0.488735 -0.48031 -0.471889 -0.463464 -0.455037 -0.446611 -0.438185 -0.429758 -0.421332 -0.412906 -0.40448 -0.396053 -0.387627 -0.370775 -0.353922 -0.337069 -0.320215 -0.303361 -0.269656 -0.235949 -0.202243 -0.168536 -0.134829 -0.101122 -0.067415 -0.033707 0 0 0 0 construction
  arc A20 (42.3328, 15.9448) -> (42.4866, 17.4115) centre (10.5928, 20.0161) ccw construction
  spline S21 degree 3 poles (42.4866, 17.4115) (42.392, 17.472) (42.2026, 17.593) (41.9132, 17.7659) (41.62, 17.9323) (41.3225, 18.0909) (41.0209, 18.2414) (40.715, 18.3831) (40.4048, 18.5151) (40.0902, 18.6364) (39.8244, 18.7274) (39.6095, 18.7932) (39.4472, 18.8385) (39.2837, 18.8798) (39.1189, 18.9148) (38.9811, 18.9426) (38.8727, 18.9722) (38.7927, 18.9988) (38.714, 19.0288) (38.637, 19.0633) (38.5625, 19.1027) (38.4909, 19.1473) (38.423, 19.1973) (38.3593, 19.2527) (38.3008, 19.3135) (38.2486, 19.3798) (38.203, 19.4508) (38.1634, 19.5253) (38.1331, 19.6041) (38.1105, 19.6854) (38.0958, 19.7685) (38.091, 19.8809) (38.094, 20.0214) (38.091, 20.1618) (38.0957, 20.2742) (38.1104, 20.3574) (38.1329, 20.4386) (38.1632, 20.5175) (38.2028, 20.592) (38.2484, 20.6629) (38.3005, 20.7293) (38.359, 20.7901) (38.4226, 20.8455) (38.4906, 20.8955) (38.5621, 20.9402) (38.6366, 20.9796) (38.7136, 21.0141) (38.7923, 21.0441) (38.8723, 21.0708) (38.9807, 21.1005) (39.1185, 21.1283) (39.2833, 21.1634) (39.4467, 21.2047) (39.609, 21.2501) (39.8239, 21.316) (40.0897, 21.4071) (40.4042, 21.5285) (40.7143, 21.6607) (41.0202, 21.8025) (41.3218, 21.9531) (41.6192, 22.1118) (41.9123, 22.2783) (42.2017, 22.4513) (42.391, 22.5724) (42.4856, 22.6329) knots -1.078574 -1.078574 -1.078574 -1.078574 -1.044867 -1.011159 -0.977452 -0.943745 -0.910038 -0.876331 -0.842624 -0.808918 -0.775212 -0.758359 -0.741505 -0.724651 -0.707798 -0.690947 -0.68252 -0.674093 -0.665668 -0.657242 -0.648815 -0.640389 -0.631963 -0.623537 -0.61511 -0.606685 -0.598264 -0.589839 -0.581413 -0.57299 -0.564565 -0.556141 -0.539287 -0.522433 -0.514009 -0.505584 -0.49716 -0.488735 -0.48031 -0.471889 -0.463464 -0.455037 -0.446611 -0.438185 -0.429758 -0.421332 -0.412906 -0.40448 -0.396053 -0.387627 -0.370775 -0.353922 -0.337069 -0.320215 -0.303361 -0.269656 -0.235949 -0.202243 -0.168536 -0.134829 -0.101122 -0.067415 -0.033707 0 0 0 0 construction
  arc A21 (42.4856, 22.6329) -> (42.3312, 24.0995) centre (10.5928, 20.0161) ccw construction
  spline S22 degree 3 poles (42.3312, 24.0995) (42.226, 24.139) (42.0156, 24.218) (41.6966, 24.327) (41.3752, 24.4287) (41.0513, 24.522) (40.7249, 24.6065) (40.3963, 24.6815) (40.0654, 24.7461) (39.7325, 24.7994) (39.4535, 24.8331) (39.2297, 24.8528) (39.0615, 24.8634) (38.893, 24.8698) (38.7245, 24.8698) (38.584, 24.8683) (38.4718, 24.8747) (38.388, 24.8842) (38.3047, 24.8971) (38.2223, 24.9148) (38.1412, 24.9379) (38.0619, 24.9667) (37.985, 25.0014) (37.9113, 25.0424) (37.8414, 25.0897) (37.7766, 25.1437) (37.7172, 25.2036) (37.663, 25.2683) (37.6169, 25.339) (37.5779, 25.4138) (37.5462, 25.4921) (37.5182, 25.6011) (37.4919, 25.7391) (37.4598, 25.8758) (37.441, 25.9867) (37.4381, 26.0711) (37.4433, 26.1553) (37.4565, 26.2387) (37.4797, 26.3199) (37.5095, 26.3987) (37.5468, 26.4745) (37.5913, 26.5461) (37.642, 26.6135) (37.6981, 26.6766) (37.7588, 26.7351) (37.8235, 26.7892) (37.8916, 26.8389) (37.9624, 26.8847) (38.035, 26.9274) (38.1349, 26.979) (38.2639, 27.0348) (38.4178, 27.1034) (38.5691, 27.1778) (38.7184, 27.256) (38.9149, 27.3651) (39.1559, 27.5094) (39.4383, 27.6936) (39.7142, 27.8873) (39.9839, 28.0896) (40.2476, 28.2997) (40.5055, 28.5168) (40.7576, 28.7405) (41.0046, 28.9699) (41.1646, 29.1277) (41.2446, 29.2066) knots -1.078574 -1.078574 -1.078574 -1.078574 -1.044867 -1.011159 -0.977452 -0.943745 -0.910038 -0.876331 -0.842624 -0.808918 -0.775212 -0.758359 -0.741505 -0.724651 -0.707798 -0.690947 -0.68252 -0.674093 -0.665668 -0.657242 -0.648815 -0.640389 -0.631963 -0.623537 -0.61511 -0.606685 -0.598264 -0.589839 -0.581413 -0.57299 -0.564565 -0.556141 -0.539287 -0.522433 -0.514009 -0.505584 -0.49716 -0.488735 -0.48031 -0.471889 -0.463464 -0.455037 -0.446611 -0.438185 -0.429758 -0.421332 -0.412906 -0.40448 -0.396053 -0.387627 -0.370775 -0.353922 -0.337069 -0.320215 -0.303361 -0.269656 -0.235949 -0.202243 -0.168536 -0.134829 -0.101122 -0.067415 -0.033707 0 0 0 0 construction
  arc A22 (41.2446, 29.2066) -> (40.7887, 30.6091) centre (10.5928, 20.0161) ccw construction
  spline S23 degree 3 poles (40.7887, 30.6091) (40.6776, 30.6258) (40.4553, 30.6593) (40.1206, 30.6996) (39.7851, 30.7323) (39.4489, 30.7562) (39.1121, 30.771) (38.775, 30.776) (38.4379, 30.7705) (38.1012, 30.7533) (37.8214, 30.7284) (37.5983, 30.701) (37.4315, 30.6764) (37.2654, 30.6477) (37.1006, 30.6127) (36.9635, 30.582) (36.8524, 30.5649) (36.7685, 30.5567) (36.6843, 30.5521) (36.6, 30.5523) (36.5159, 30.558) (36.4323, 30.5696) (36.3499, 30.5877) (36.2693, 30.6124) (36.1911, 30.6441) (36.1164, 30.6835) (36.0459, 30.7297) (35.9794, 30.7817) (35.9197, 30.8413) (35.866, 30.9064) (35.8187, 30.9764) (35.7687, 31.0772) (35.7143, 31.2066) (35.6544, 31.3337) (35.613, 31.4383) (35.5925, 31.5203) (35.5801, 31.6037) (35.5757, 31.688) (35.5815, 31.7722) (35.5943, 31.8555) (35.615, 31.9374) (35.6437, 32.0167) (35.6793, 32.0932) (35.721, 32.1665) (35.7682, 32.2364) (35.8202, 32.3028) (35.8765, 32.3656) (35.9362, 32.425) (35.9984, 32.482) (36.0854, 32.5531) (36.1999, 32.6345) (36.3362, 32.7337) (36.4687, 32.8379) (36.5985, 32.9454) (36.768, 33.093) (36.9738, 33.2843) (37.2117, 33.5232) (37.4413, 33.77) (37.663, 34.0239) (37.8773, 34.2842) (38.0844, 34.5502) (38.2845, 34.8215) (38.4784, 35.0972) (38.6022, 35.2848) (38.664, 35.3786) knots -1.078574 -1.078574 -1.078574 -1.078574 -1.044867 -1.011159 -0.977452 -0.943745 -0.910038 -0.876331 -0.842624 -0.808918 -0.775212 -0.758359 -0.741505 -0.724651 -0.707798 -0.690947 -0.68252 -0.674093 -0.665668 -0.657242 -0.648815 -0.640389 -0.631963 -0.623537 -0.61511 -0.606685 -0.598264 -0.589839 -0.581413 -0.57299 -0.564565 -0.556141 -0.539287 -0.522433 -0.514009 -0.505584 -0.49716 -0.488735 -0.48031 -0.471889 -0.463464 -0.455037 -0.446611 -0.438185 -0.429758 -0.421332 -0.412906 -0.40448 -0.396053 -0.387627 -0.370775 -0.353922 -0.337069 -0.320215 -0.303361 -0.269656 -0.235949 -0.202243 -0.168536 -0.134829 -0.101122 -0.067415 -0.033707 0 0 0 0 construction
  arc A23 (38.664, 35.3786) -> (37.9264, 36.6557) centre (10.5928, 20.0161) ccw construction